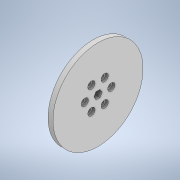
# Autodesk Inventor part: halfWheelForHangingAndMovingV2
Saved by Autodesk Inventor 2020.2 (Build 242310000, 310)
## iProperties
Created: 2020-01-09
Part Number: halfWheelForHangingAndMovingV2
Material: Generic
Document SubType Name: Modeling
Designer: robst
Density: 1 g/cm^3
Appearance: Default
Author: robst
Autodesk Inventor part; units mm, degrees
ref_plane "YZ Plane" through (0, 0, 0) normal (1, 0, 0) x (0, 1, 0)
ref_plane "XZ Plane" through (0, 0, 0) normal (0, 1, 0) x (-1, 0, 0)
ref_plane "XY Plane" through (0, 0, 0) normal (0, 0, 1) x (1, 0, 0)
sketch "Sketch1" plane through (0, 0, 0) normal (0, 0, 1) x (1, 0, 0)
  arc A0 (0, 31.75) -> (21.1582, 52.9082) centre (0, 52.9082) ccw
  line L0 (0, 31.75) -> (38.8128, 31.75) construction
  line L1 (30.6832, 0) -> (30.6832, 86.3474)
  line L2 (21.1582, 52.9082) -> (21.1582, 86.3474)
  line L3 (21.1582, 86.3474) -> (30.6832, 86.3474)
  line L4 (0, 79.9974) -> (0, 0) construction
  line L5 (0, 31.75) -> (0, 0)
  line L6 (30.6832, 0) -> (0, 0)
  dimension "pipeDiameter" = 42.3164
  dimension "d1" = 31.75
  dimension "width" = 9.525
  constraints: 14 end point, 3 vertical, 2 horizontal, 2 point on circle, 2 tangent, 1 centre point, 1 perpendicular
  measures "pipeDiameter" diameter of A0
  measures "d1" distance from line of L4.end L0
  measures "width" distance between parallel lines of L1 L2
revolve "Revolution1" add sketch "Sketch1" angle 360 about axis through (30.6832, 0, 0) along (-1, 0, 0)
sketch "Sketch2" plane through (30.6832, 0, 0) normal (1, 0, 0) x (0, 0, -1)
  line L0 (-3.9595, 6.858) -> (3.9595, 6.858)
  line L1 (3.9595, 6.858) -> (7.9189, 0)
  line L2 (7.9189, 0) -> (3.9595, -6.858)
  line L3 (3.9595, -6.858) -> (-3.9595, -6.858)
  line L4 (-3.9595, -6.858) -> (-7.9189, 0)
  line L5 (-7.9189, 0) -> (-3.9595, 6.858)
  point P0 (0, 0)
  point P1 (0, 0)
  dimension "hexWidth" = 13.716
  constraints: 12 end point, 1 coincident, 1 horizontal, 13 other
  measures "hexWidth" distance between parallel lines of L0 L3
extrude "Extrusion1" cut sketch "Sketch2" against normal through all
sketch "Sketch3" plane through (30.6832, 0, 0) normal (1, 0, 0) x (0, 0, -1)
  point P0 (0, 0)
  point P1 (-25.4, 0)
  point P2 (-12.7, -21.997)
  point P3 (12.7, -21.997)
  point P4 (25.4, 0)
  point P5 (12.7, 21.997)
  point P6 (-12.7, 21.997)
  dimension "d7" = 25.4
  dimension "d10" = 360
  constraints: 7 other
  measures "d7" distance of point (-25.4, 0) point (0, 0)
hole "Hole1" at (30.6832, 0, 25.4) at (30.6832, -21.997, 12.7) at (30.6832, -21.997, -12.7) at (30.6832, 0, -25.4) at (30.6832, 21.997, -12.7) at (30.6832, 21.997, 12.7) direction (-1, 0, 0) diameter 6.7564 end through all counterbore diameter 13.97 counterbore depth 4.7752 clearance for "Hex Head Bolt" size "1/4" standard "Ansi Unified Screw Threads"
body "Solid1"
